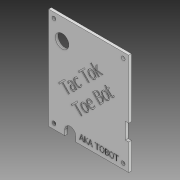
# Autodesk Inventor part: Electronics Lid
Saved by Autodesk Inventor 2020 (Build 240168000, 168)
## iProperties
Created: 2020-09-05
Part Number: Electronics Lid
Material: Generic
Document SubType Name: Modeling
Designer: DDeGo
Density: 1 g/cm^3
Appearance: Default
Author: DDeGo
Autodesk Inventor part; units mm, degrees
ref_plane "YZ Plane" through (0, 0, 0) normal (1, 0, 0) x (0, 1, 0)
ref_plane "XZ Plane" through (0, 0, 0) normal (0, 1, 0) x (-1, 0, 0)
ref_plane "XY Plane" through (0, 0, 0) normal (0, 0, 1) x (1, 0, 0)
sketch "Sketch1" plane through (0, 0, 0) normal (0, 0, 1) x (1, 0, 0)
  line L0 (-37, -47) -> (37, -47)
  line L1 (37, -47) -> (37, 47)
  line L2 (37, 47) -> (-37, 47)
  line L3 (-37, 47) -> (-37, -47)
  line L4 (-37, -47) -> (37, 47) construction
  line L5 (37, -47) -> (-37, 47) construction
  line L6 (-32, -42) -> (32, -42) construction
  line L7 (32, -42) -> (32, 42) construction
  line L8 (32, 42) -> (-32, 42) construction
  line L9 (-32, 42) -> (-32, -42) construction
  line L10 (-32, -42) -> (32, 42) construction
  line L11 (32, -42) -> (-32, 42) construction
  circle A0 centre (-32, 42) radius 1.75
  circle A1 centre (32, 42) radius 1.75
  circle A2 centre (32, -42) radius 1.75
  circle A3 centre (-32, -42) radius 1.75
  point P0 (0, 0)
  dimension "d0" = 74
  dimension "d1" = 94
  dimension "d2" = 84
  dimension "d3" = 64
  dimension "d4" = 3.5
  constraints: 24 end point, 4 centre point, 4 coincident, 4 midpoint, 4 parallel, 3 equal radius, 2 horizontal, 2 perpendicular
  measures "d0" distance of L1.end L2.end
  measures "d1" distance of L0.end L1.end
  measures "d2" distance of L6.end L7.end
  measures "d3" distance of L7.end L8.end
  measures "d4" diameter of A0
extrude "Extrusion1" add sketch "Sketch1" along normal blind 2.5
sketch "Sketch2" plane through (0, 0, 2.5) normal (0, 0, 1) x (1, 0, 0)
  line L0 (37, -47) -> (37, 47) projected
  line L1 (37, -22.5) -> (34, -22.5)
  line L2 (34, -22.5) -> (34, -7.5)
  line L3 (34, -7.5) -> (37, -7.5)
  line L4 (37, -7.5) -> (37, -22.5)
  circle A0 centre (32, -42) radius 1.75 projected
  circle A1 centre (-24.5, 27.5) radius 6.25
  line L5 (37, 47) -> (-37, 47) projected
  line L6 (-37, 47) -> (-37, -47) projected
  arc A2 (-12, -42) -> (-22, -42) centre (-17, -42) ccw
  line L7 (-22, -42) -> (-22, -47)
  line L8 (-37, -47) -> (37, -47) projected
  line L9 (-22, -47) -> (-12, -47)
  line L10 (-12, -47) -> (-12, -42)
  circle A3 centre (-32, -42) radius 1.75 projected
  point P0 (0, 0)
  point P1 (34, -15)
  dimension "d7" = 27
  dimension "d8" = 15
  dimension "d9" = 3
  dimension "d10" = 19.5
  dimension "d11" = 12.5
  dimension "d12" = 12.5
  dimension "d13" = 5
  dimension "d14" = 5
  dimension "d15" = 15
  constraints: 14 end point, 2 centre point, 2 horizontal, 2 parallel, 2 point on circle, 2 point on line, 2 tangent, 2 vertical, 1 midpoint, 1 perpendicular
  measures "d7" vertical distance of A0.centre point (34, -15)
  measures "d8" distance of L1.end L2.end
  measures "d9" distance of L1.start L1.end
  measures "d10" distance from line of L5 A1.centre
  measures "d11" distance from line of L6 A1.centre
  measures "d12" diameter of A1
  measures "d13" radius of A2
  measures "d14" distance from line of L8 A2.centre
  measures "d15" distance of A3.centre A2.centre
extrude "Extrusion2" cut sketch "Sketch2" against normal through all contours L1 L2 L3 L0 | L8 L7 A2 L10 | A0 | A1 | A3
sketch "Sketch3" plane through (0, 0, 2.5) normal (0, 0, 1) x (1, 0, 0)
  line L0 (-28.3077, -7.093) -> (10.2074, 31.4221) construction
  line L1 (10.2074, 31.4221) -> (33.5157, 8.1138) construction
  line L2 (33.5157, 8.1138) -> (-4.9994, -30.4013) construction
  line L3 (-4.9994, -30.4013) -> (-28.3077, -7.093) construction
  line L4 (-12, -47) -> (37, -47) projected
  line L5 (-8.6021, -38.2619) -> (27.6581, -38.2619) construction
  line L6 (27.6581, -38.2619) -> (27.6581, -43.4725) construction
  line L7 (27.6581, -43.4725) -> (-8.6021, -43.4725) construction
  line L8 (-8.6021, -43.4725) -> (-8.6021, -38.2619) construction
  line L9 (-18.5549, -12.1126) -> (-24.7894, -5.8782)
  line L10 (-24.7894, -5.8782) -> (-27.1617, -8.2505)
  line L11 (-27.1617, -8.2505) -> (-27.9983, -7.4139)
  line L12 (-27.9983, -7.4139) -> (-22.3139, -1.7295)
  line L13 (-22.3139, -1.7295) -> (-21.4773, -2.5661)
  line L14 (-21.4773, -2.5661) -> (-23.8496, -4.9384)
  line L15 (-23.8496, -4.9384) -> (-17.6151, -11.1729)
  line L16 (-17.6151, -11.1729) -> (-18.5549, -12.1126)
  spline S0 degree 2 poles (-12.2001, -4.6347) (-12.2288, -4.8238) (-12.309, -5.4771) (-12.3949, -5.7349) knots 0 0 0 1 2 2 2
  spline S1 degree 2 poles (-12.3949, -5.7349) (-12.5038, -6.0959) (-12.8132, -6.6689) (-13.2144, -7.0701) knots 0 0 0 1 2 2 2
  spline S2 degree 2 poles (-13.2144, -7.0701) (-13.541, -7.3967) (-14.3776, -7.7405) (-14.8245, -7.7405) knots 0 0 0 1 2 2 2
  spline S3 degree 2 poles (-14.8245, -7.7405) (-15.2543, -7.7348) (-16.1539, -7.3508) (-16.5092, -6.9956) knots 0 0 0 1 2 2 2
  spline S4 degree 2 poles (-16.5092, -6.9956) (-17.0593, -6.4455) (-17.3745, -5.202) (-17.0937, -4.4743) knots 0 0 0 1 2 2 2
  spline S5 degree 2 poles (-17.0937, -4.4743) (-16.853, -3.821) (-15.7929, -2.4515) (-15.1282, -1.7066) knots 0 0 0 1 2 2 2
  line L17 (-15.1282, -1.7066) -> (-15.3001, -1.5347)
  spline S6 degree 2 poles (-15.3001, -1.5347) (-15.6096, -1.2253) (-16.1826, -1.0304) (-16.4634, -1.0935) knots 0 0 0 1 2 2 2
  spline S7 degree 2 poles (-16.4634, -1.0935) (-16.7442, -1.1565) (-17.3057, -1.5805) (-17.5693, -1.8441) knots 0 0 0 1 2 2 2
  spline S8 degree 2 poles (-17.5693, -1.8441) (-17.8787, -2.1535) (-18.532, -3.1735) (-18.7726, -3.7695) knots 0 0 0 1 2 2 2
  line L18 (-18.7726, -3.7695) -> (-18.8242, -3.821)
  line L19 (-18.8242, -3.821) -> (-19.7353, -2.9099)
  spline S9 degree 2 poles (-19.7353, -2.9099) (-19.5577, -2.5948) (-18.807, -1.5003) (-18.3543, -1.0476) knots 0 0 0 1 2 2 2
  spline S10 degree 2 poles (-18.3543, -1.0476) (-17.8042, -0.4975) (-16.8817, 0.0812) (-16.3602, 0.1557) knots 0 0 0 1 2 2 2
  spline S11 degree 2 poles (-16.3602, 0.1557) (-15.8502, 0.2302) (-14.8704, -0.1766) (-14.3719, -0.6752) knots 0 0 0 1 2 2 2
  line L20 (-14.3719, -0.6752) -> (-10.7446, -4.3024)
  line L21 (-10.7446, -4.3024) -> (-11.6385, -5.1963)
  line L22 (-11.6385, -5.1963) -> (-12.2001, -4.6347)
  line L23 (-12.945, -3.8898) -> (-14.4177, -2.4171)
  spline S12 degree 2 poles (-14.4177, -2.4171) (-14.7099, -2.7667) (-15.5809, -3.8325) (-15.7929, -4.2279) knots 0 0 0 1 2 2 2
  spline S13 degree 2 poles (-15.7929, -4.2279) (-16.0393, -4.692) (-16.0508, -5.6089) (-15.6497, -6.01) knots 0 0 0 1 2 2 2
  spline S14 degree 2 poles (-15.6497, -6.01) (-15.1913, -6.4684) (-14.2114, -6.4168) (-13.7186, -5.924) knots 0 0 0 1 2 2 2
  spline S15 degree 2 poles (-13.7186, -5.924) (-13.3003, -5.5057) (-12.9737, -4.4571) (-12.945, -3.8898) knots 0 0 0 1 2 2 2
  spline S16 degree 2 poles (-7.2607, -1.0591) (-7.8108, -1.6092) (-9.06, -2.1822) (-9.7304, -2.165) knots 0 0 0 1 2 2 2
  spline S17 degree 2 poles (-9.7304, -2.165) (-10.3951, -2.1535) (-11.799, -1.4717) (-12.4981, -0.7726) knots 0 0 0 1 2 2 2
  spline S18 degree 2 poles (-12.4981, -0.7726) (-13.1972, -0.0735) (-13.8447, 1.319) (-13.8733, 1.9779) knots 0 0 0 1 2 2 2
  spline S19 degree 2 poles (-13.8733, 1.9779) (-13.9077, 2.6426) (-13.3461, 3.9491) (-12.8075, 4.4878) knots 0 0 0 1 2 2 2
  spline S20 degree 2 poles (-12.8075, 4.4878) (-12.372, 4.9233) (-11.3119, 5.4905) (-10.8363, 5.6453) knots 0 0 0 1 2 2 2
  line L24 (-10.8363, 5.6453) -> (-9.8335, 4.6425)
  line L25 (-9.8335, 4.6425) -> (-9.8851, 4.5909)
  spline S21 degree 2 poles (-9.8851, 4.5909) (-10.0627, 4.5737) (-10.567, 4.482) (-10.8879, 4.3789) knots 0 0 0 1 2 2 2
  spline S22 degree 2 poles (-10.8879, 4.3789) (-11.1687, 4.2815) (-11.8162, 3.9205) (-12.0454, 3.6913) knots 0 0 0 1 2 2 2
  spline S23 degree 2 poles (-12.0454, 3.6913) (-12.7387, 2.9979) (-12.5325, 1.1069) (-11.5755, 0.15) knots 0 0 0 1 2 2 2
  spline S24 degree 2 poles (-11.5755, 0.15) (-10.6415, -0.784) (-8.7792, -1.019) (-8.0572, -0.297) knots 0 0 0 1 2 2 2
  spline S25 degree 2 poles (-8.0572, -0.297) (-7.6217, 0.1385) (-7.1919, 1.2903) (-7.169, 1.8748) knots 0 0 0 1 2 2 2
  line L26 (-7.169, 1.8748) -> (-7.1174, 1.9264)
  line L27 (-7.1174, 1.9264) -> (-6.1146, 0.9236)
  spline S26 degree 2 poles (-6.1146, 0.9236) (-6.1834, 0.7287) (-6.4069, 0.15) (-6.5272, -0.0506) knots 0 0 0 1 2 2 2
  spline S27 degree 2 poles (-6.5272, -0.0506) (-6.6877, -0.3485) (-6.9799, -0.7783) (-7.2607, -1.0591) knots 0 0 0 1 2 2 2
  line L28 (-0.2469, 6.1954) -> (-6.4814, 12.4298)
  line L29 (-6.4814, 12.4298) -> (-8.8537, 10.0575)
  line L30 (-8.8537, 10.0575) -> (-9.6903, 10.8941)
  line L31 (-9.6903, 10.8941) -> (-4.0059, 16.5785)
  line L32 (-4.0059, 16.5785) -> (-3.1693, 15.7419)
  line L33 (-3.1693, 15.7419) -> (-5.5416, 13.3696)
  line L34 (-5.5416, 13.3696) -> (0.6928, 7.1351)
  line L35 (0.6928, 7.1351) -> (-0.2469, 6.1954)
  spline S28 degree 2 poles (5.4203, 17.1687) (6.7611, 15.8278) (6.933, 13.0773) (5.8558, 12) knots 0 0 0 1 2 2 2
  spline S29 degree 2 poles (5.8558, 12) (4.7498, 10.8941) (1.9764, 11.1348) (0.6814, 12.4298) knots 0 0 0 1 2 2 2
  spline S30 degree 2 poles (0.6814, 12.4298) (-0.648, 13.7592) (-0.8142, 16.5384) (0.2516, 17.6042) knots 0 0 0 1 2 2 2
  spline S31 degree 2 poles (0.2516, 17.6042) (1.3289, 18.6815) (4.0851, 18.5038) (5.4203, 17.1687) knots 0 0 0 1 2 2 2
  spline S32 degree 2 poles (4.4977, 16.2461) (3.4663, 17.2776) (1.7128, 17.5297) (1.0195, 16.8363) knots 0 0 0 1 2 2 2
  spline S33 degree 2 poles (1.0195, 16.8363) (0.3261, 16.143) (0.5725, 14.3838) (1.6039, 13.3524) knots 0 0 0 1 2 2 2
  spline S34 degree 2 poles (1.6039, 13.3524) (2.6067, 12.3496) (4.3946, 12.0745) (5.0879, 12.7679) knots 0 0 0 1 2 2 2
  spline S35 degree 2 poles (5.0879, 12.7679) (5.7755, 13.4555) (5.5177, 15.2262) (4.4977, 16.2461) knots 0 0 0 1 2 2 2
  line L36 (13.3852, 19.8275) -> (12.2105, 18.6528)
  line L37 (12.2105, 18.6528) -> (7.678, 19.243)
  line L38 (7.678, 19.243) -> (7.6665, 18.5439)
  line L39 (7.6665, 18.5439) -> (9.8841, 16.3264)
  line L40 (9.8841, 16.3264) -> (8.9902, 15.4324)
  line L41 (8.9902, 15.4324) -> (1.6039, 22.8187)
  line L42 (1.6039, 22.8187) -> (2.4979, 23.7126)
  line L43 (2.4979, 23.7126) -> (6.8184, 19.392)
  line L44 (6.8184, 19.392) -> (6.6752, 23.7298)
  line L45 (6.6752, 23.7298) -> (7.7868, 24.8414)
  line L46 (7.7868, 24.8414) -> (7.8269, 20.4464)
  line L47 (7.8269, 20.4464) -> (13.3852, 19.8275)
  line L48 (-6.9126, -23.755) -> (-13.147, -17.5205)
  line L49 (-13.147, -17.5205) -> (-15.5193, -19.8928)
  line L50 (-15.5193, -19.8928) -> (-16.3559, -19.0562)
  line L51 (-16.3559, -19.0562) -> (-10.6716, -13.3718)
  line L52 (-10.6716, -13.3718) -> (-9.835, -14.2084)
  line L53 (-9.835, -14.2084) -> (-12.2073, -16.5808)
  line L54 (-12.2073, -16.5808) -> (-5.9728, -22.8152)
  line L55 (-5.9728, -22.8152) -> (-6.9126, -23.755)
  spline S36 degree 2 poles (-1.2454, -12.7816) (0.0955, -14.1225) (0.2674, -16.873) (-0.8099, -17.9503) knots 0 0 0 1 2 2 2
  spline S37 degree 2 poles (-0.8099, -17.9503) (-1.9158, -19.0562) (-4.6893, -18.8155) (-5.9843, -17.5205) knots 0 0 0 1 2 2 2
  spline S38 degree 2 poles (-5.9843, -17.5205) (-7.3137, -16.1911) (-7.4799, -13.412) (-6.414, -12.3461) knots 0 0 0 1 2 2 2
  spline S39 degree 2 poles (-6.414, -12.3461) (-5.3368, -11.2689) (-2.5805, -11.4465) (-1.2454, -12.7816) knots 0 0 0 1 2 2 2
  spline S40 degree 2 poles (-2.168, -13.7042) (-3.1994, -12.6728) (-4.9528, -12.4206) (-5.6462, -13.114) knots 0 0 0 1 2 2 2
  spline S41 degree 2 poles (-5.6462, -13.114) (-6.3396, -13.8073) (-6.0932, -15.5665) (-5.0617, -16.5979) knots 0 0 0 1 2 2 2
  spline S42 degree 2 poles (-5.0617, -16.5979) (-4.0589, -17.6007) (-2.2711, -17.8758) (-1.5778, -17.1824) knots 0 0 0 1 2 2 2
  spline S43 degree 2 poles (-1.5778, -17.1824) (-0.8901, -16.4948) (-1.148, -14.7242) (-2.168, -13.7042) knots 0 0 0 1 2 2 2
  spline S44 degree 2 poles (4.7484, -12.3347) (3.4763, -13.6068) (0.6513, -13.5781) (-0.6667, -12.2602) knots 0 0 0 1 2 2 2
  spline S45 degree 2 poles (-0.6667, -12.2602) (-1.9617, -10.9652) (-2.1393, -8.0714) (-1.0448, -6.9769) knots 0 0 0 1 2 2 2
  spline S46 degree 2 poles (-1.0448, -6.9769) (-0.5521, -6.4841) (0.4966, -6.0085) (1.0811, -6.0315) knots 0 0 0 1 2 2 2
  spline S47 degree 2 poles (1.0811, -6.0315) (1.6713, -6.0486) (2.8517, -6.6217) (3.4877, -7.2577) knots 0 0 0 1 2 2 2
  line L56 (3.4877, -7.2577) -> (3.9748, -7.7448)
  line L57 (3.9748, -7.7448) -> (0.3017, -11.4178)
  spline S48 degree 2 poles (0.3017, -11.4178) (1.2243, -12.3404) (3.1325, -12.392) (3.9576, -11.5668) knots 0 0 0 1 2 2 2
  spline S49 degree 2 poles (3.9576, -11.5668) (4.2499, -11.2746) (4.6854, -10.5755) (4.8114, -10.2431) knots 0 0 0 1 2 2 2
  spline S50 degree 2 poles (4.8114, -10.2431) (4.9375, -9.8879) (5.0693, -9.355) (5.0865, -9.1544) knots 0 0 0 1 2 2 2
  line L58 (5.0865, -9.1544) -> (5.138, -9.1028)
  line L59 (5.138, -9.1028) -> (6.1122, -10.077)
  spline S51 degree 2 poles (6.1122, -10.077) (6.0205, -10.2947) (5.734, -10.948) (5.6022, -11.1829) knots 0 0 0 1 2 2 2
  spline S52 degree 2 poles (5.6022, -11.1829) (5.4188, -11.5153) (5.0693, -12.0138) (4.7484, -12.3347) knots 0 0 0 1 2 2 2
  spline S53 degree 2 poles (2.4219, -7.9339) (2.0495, -7.5843) (1.3733, -7.2061) (1.0524, -7.1718) knots 0 0 0 1 2 2 2
  spline S54 degree 2 poles (1.0524, -7.1718) (0.6971, -7.1259) (-0.002, -7.401) (-0.363, -7.762) knots 0 0 0 1 2 2 2
  spline S55 degree 2 poles (-0.363, -7.762) (-0.7182, -8.1172) (-1.0047, -8.8278) (-1.0047, -9.2404) knots 0 0 0 1 2 2 2
  spline S56 degree 2 poles (-1.0047, -9.2404) (-0.9933, -9.6529) (-0.6896, -10.3692) (-0.3801, -10.7359) knots 0 0 0 1 2 2 2
  line L60 (-0.3801, -10.7359) -> (2.4219, -7.9339)
  spline S57 degree 2 poles (13.1718, 0.6729) (13.699, 0.1457) (14.1058, -1.0634) (14.037, -1.6593) knots 0 0 0 1 2 2 2
  spline S58 degree 2 poles (14.037, -1.6593) (13.9454, -2.3699) (13.2978, -3.5445) (12.5758, -4.2665) knots 0 0 0 1 2 2 2
  line L61 (12.5758, -4.2665) -> (10.5473, -6.295)
  line L62 (10.5473, -6.295) -> (3.4763, 0.776)
  line L63 (3.4763, 0.776) -> (5.3501, 2.6498)
  spline S59 degree 2 poles (5.3501, 2.6498) (6.1064, 3.4062) (6.9602, 4.0652) (7.4932, 4.2199) knots 0 0 0 1 2 2 2
  spline S60 degree 2 poles (7.4932, 4.2199) (8.0776, 4.4032) (9.0861, 4.0938) (9.5331, 3.6469) knots 0 0 0 1 2 2 2
  spline S61 degree 2 poles (9.5331, 3.6469) (10.0316, 3.1483) (10.2952, 1.8304) (10.0546, 1.1428) knots 0 0 0 1 2 2 2
  line L64 (10.0546, 1.1428) -> (10.0889, 1.1084)
  spline S62 degree 2 poles (10.0889, 1.1084) (10.8912, 1.5668) (12.4956, 1.349) (13.1718, 0.6729) knots 0 0 0 1 2 2 2
  spline S63 degree 2 poles (12.232, -0.3471) (11.8309, 0.054) (11.086, 0.3405) (10.5588, 0.1801) knots 0 0 0 1 2 2 2
  spline S64 degree 2 poles (10.5588, 0.1801) (10.2207, 0.0712) (9.6248, -0.3872) (9.1377, -0.8743) knots 0 0 0 1 2 2 2
  line L65 (9.1377, -0.8743) -> (8.0719, -1.9401)
  line L66 (8.0719, -1.9401) -> (10.6849, -4.5531)
  line L67 (10.6849, -4.5531) -> (11.447, -3.7909)
  spline S65 degree 2 poles (11.447, -3.7909) (12.0659, -3.1721) (12.6618, -2.3469) (12.7535, -1.8885) knots 0 0 0 1 2 2 2
  spline S66 degree 2 poles (12.7535, -1.8885) (12.828, -1.4358) (12.6045, -0.7196) (12.232, -0.3471) knots 0 0 0 1 2 2 2
  spline S67 degree 2 poles (8.685, 2.5352) (8.4329, 2.7873) (7.8828, 2.9936) (7.5848, 2.9134) knots 0 0 0 1 2 2 2
  spline S68 degree 2 poles (7.5848, 2.9134) (7.2296, 2.8102) (6.6164, 2.3117) (6.1179, 1.8132) knots 0 0 0 1 2 2 2
  line L68 (6.1179, 1.8132) -> (5.2183, 0.9136)
  line L69 (5.2183, 0.9136) -> (7.2869, -1.1551)
  line L70 (7.2869, -1.1551) -> (8.3527, -0.0892)
  spline S69 degree 2 poles (8.3527, -0.0892) (8.7939, 0.352) (9.1205, 0.862) (9.2008, 1.2287) knots 0 0 0 1 2 2 2
  spline S70 degree 2 poles (9.2008, 1.2287) (9.281, 1.584) (9.0174, 2.2028) (8.685, 2.5352) knots 0 0 0 1 2 2 2
  spline S71 degree 2 poles (17.9164, 6.3802) (19.2573, 5.0393) (19.4292, 2.2888) (18.3519, 1.2115) knots 0 0 0 1 2 2 2
  spline S72 degree 2 poles (18.3519, 1.2115) (17.246, 0.1056) (14.4725, 0.3463) (13.1775, 1.6413) knots 0 0 0 1 2 2 2
  spline S73 degree 2 poles (13.1775, 1.6413) (11.8481, 2.9707) (11.6819, 5.7498) (12.7477, 6.8157) knots 0 0 0 1 2 2 2
  spline S74 degree 2 poles (12.7477, 6.8157) (13.825, 7.8929) (16.5812, 7.7153) (17.9164, 6.3802) knots 0 0 0 1 2 2 2
  spline S75 degree 2 poles (16.9938, 5.4576) (15.9624, 6.489) (14.2089, 6.7412) (13.5156, 6.0478) knots 0 0 0 1 2 2 2
  spline S76 degree 2 poles (13.5156, 6.0478) (12.8222, 5.3545) (13.0686, 3.5953) (14.1001, 2.5638) knots 0 0 0 1 2 2 2
  spline S77 degree 2 poles (14.1001, 2.5638) (15.1029, 1.5611) (16.8907, 1.286) (17.584, 1.9794) knots 0 0 0 1 2 2 2
  spline S78 degree 2 poles (17.584, 1.9794) (18.2717, 2.667) (18.0138, 4.4376) (16.9938, 5.4576) knots 0 0 0 1 2 2 2
  spline S79 degree 2 poles (23.1939, 6.1452) (22.4662, 5.4175) (20.8159, 5.429) (19.9162, 6.3286) knots 0 0 0 1 2 2 2
  line L71 (19.9162, 6.3286) -> (16.9766, 9.2682)
  line L72 (16.9766, 9.2682) -> (16.375, 8.6665)
  line L73 (16.375, 8.6665) -> (15.6358, 9.4057)
  line L74 (15.6358, 9.4057) -> (16.2374, 10.0074)
  line L75 (16.2374, 10.0074) -> (14.7132, 11.5316)
  line L76 (14.7132, 11.5316) -> (15.6071, 12.4255)
  line L77 (15.6071, 12.4255) -> (17.1313, 10.9013)
  line L78 (17.1313, 10.9013) -> (18.7759, 12.5459)
  line L79 (18.7759, 12.5459) -> (19.5151, 11.8067)
  line L80 (19.5151, 11.8067) -> (17.8705, 10.1621)
  line L81 (17.8705, 10.1621) -> (20.3976, 7.6351)
  spline S80 degree 2 poles (20.3976, 7.6351) (20.7987, 7.234) (21.2686, 6.8214) (21.5551, 6.7297) knots 0 0 0 1 2 2 2
  spline S81 degree 2 poles (21.5551, 6.7297) (21.8015, 6.6438) (22.3286, 6.8386) (22.6381, 7.148) knots 0 0 0 1 2 2 2
  spline S82 degree 2 poles (22.6381, 7.148) (22.8558, 7.3658) (23.1309, 7.9044) (23.1824, 8.0362) knots 0 0 0 1 2 2 2
  line L82 (23.1824, 8.0362) -> (23.234, 8.0878)
  line L83 (23.234, 8.0878) -> (24.0362, 7.2855)
  spline S83 degree 2 poles (24.0362, 7.2855) (23.8529, 6.9646) (23.4174, 6.3687) (23.1939, 6.1452) knots 0 0 0 1 2 2 2
  line L84 (-8.6345, -43.3672) -> (-6.9489, -38.3672)
  line L85 (-6.9489, -38.3672) -> (-6.1304, -38.3672)
  line L86 (-6.1304, -38.3672) -> (-4.4448, -43.3672)
  line L87 (-4.4448, -43.3672) -> (-5.1458, -43.3672)
  line L88 (-5.1458, -43.3672) -> (-5.5996, -41.9693)
  line L89 (-5.5996, -41.9693) -> (-7.5081, -41.9693)
  line L90 (-7.5081, -41.9693) -> (-7.9619, -43.3672)
  line L91 (-7.9619, -43.3672) -> (-8.6345, -43.3672)
  line L92 (-5.782, -41.402) -> (-6.5559, -39.0479)
  line L93 (-6.5559, -39.0479) -> (-7.3257, -41.402)
  line L94 (-7.3257, -41.402) -> (-5.782, -41.402)
  line L95 (-0.3241, -43.3672) -> (-1.1871, -43.3672)
  line L96 (-1.1871, -43.3672) -> (-3.0145, -41.0414)
  line L97 (-3.0145, -41.0414) -> (-3.3063, -41.3696)
  line L98 (-3.3063, -41.3696) -> (-3.3063, -43.3672)
  line L99 (-3.3063, -43.3672) -> (-3.9708, -43.3672)
  line L100 (-3.9708, -43.3672) -> (-3.9708, -38.3672)
  line L101 (-3.9708, -38.3672) -> (-3.3063, -38.3672)
  line L102 (-3.3063, -38.3672) -> (-3.3063, -40.6646)
  line L103 (-3.3063, -40.6646) -> (-1.256, -38.3672)
  line L104 (-1.256, -38.3672) -> (-0.4457, -38.3672)
  line L105 (-0.4457, -38.3672) -> (-2.5162, -40.5998)
  line L106 (-2.5162, -40.5998) -> (-0.3241, -43.3672)
  line L107 (-0.4659, -43.3672) -> (1.2197, -38.3672)
  line L108 (1.2197, -38.3672) -> (2.0381, -38.3672)
  line L109 (2.0381, -38.3672) -> (3.7237, -43.3672)
  line L110 (3.7237, -43.3672) -> (3.0227, -43.3672)
  line L111 (3.0227, -43.3672) -> (2.5689, -41.9693)
  line L112 (2.5689, -41.9693) -> (0.6605, -41.9693)
  line L113 (0.6605, -41.9693) -> (0.2067, -43.3672)
  line L114 (0.2067, -43.3672) -> (-0.4659, -43.3672)
  line L115 (2.3866, -41.402) -> (1.6127, -39.0479)
  line L116 (1.6127, -39.0479) -> (0.8428, -41.402)
  line L117 (0.8428, -41.402) -> (2.3866, -41.402)
  line L118 (7.5122, -43.3672) -> (7.5122, -38.9588)
  line L119 (7.5122, -38.9588) -> (5.8347, -38.9588)
  line L120 (5.8347, -38.9588) -> (5.8347, -38.3672)
  line L121 (5.8347, -38.3672) -> (9.8542, -38.3672)
  line L122 (9.8542, -38.3672) -> (9.8542, -38.9588)
  line L123 (9.8542, -38.9588) -> (8.1767, -38.9588)
  line L124 (8.1767, -38.9588) -> (8.1767, -43.3672)
  line L125 (8.1767, -43.3672) -> (7.5122, -43.3672)
  spline S84 degree 2 poles (13.8979, -38.9385) (14.1816, -39.2708) (14.4976, -40.2432) (14.4976, -40.8672) knots 0 0 0 1 2 2 2
  spline S85 degree 2 poles (14.4976, -40.8672) (14.4976, -41.475) (14.1897, -42.4596) (13.8979, -42.7918) knots 0 0 0 1 2 2 2
  spline S86 degree 2 poles (13.8979, -42.7918) (13.59, -43.1403) (12.7756, -43.4725) (12.2853, -43.4725) knots 0 0 0 1 2 2 2
  spline S87 degree 2 poles (12.2853, -43.4725) (11.7788, -43.4725) (10.9684, -43.1281) (10.6727, -42.7918) knots 0 0 0 1 2 2 2
  spline S88 degree 2 poles (10.6727, -42.7918) (10.385, -42.4596) (10.077, -41.4831) (10.077, -40.8672) knots 0 0 0 1 2 2 2
  spline S89 degree 2 poles (10.077, -40.8672) (10.077, -40.2392) (10.389, -39.2829) (10.6767, -38.9385) knots 0 0 0 1 2 2 2
  spline S90 degree 2 poles (10.6767, -38.9385) (10.9684, -38.6063) (11.7829, -38.2619) (12.2853, -38.2619) knots 0 0 0 1 2 2 2
  spline S91 degree 2 poles (12.2853, -38.2619) (12.7958, -38.2619) (13.6143, -38.6184) (13.8979, -38.9385) knots 0 0 0 1 2 2 2
  spline S92 degree 2 poles (13.8048, -40.8672) (13.8048, -40.3729) (13.59, -39.6071) (13.3955, -39.3559) knots 0 0 0 1 2 2 2
  spline S93 degree 2 poles (13.3955, -39.3559) (13.197, -39.0965) (12.6378, -38.8372) (12.2894, -38.8372) knots 0 0 0 1 2 2 2
  spline S94 degree 2 poles (12.2894, -38.8372) (11.9287, -38.8372) (11.3858, -39.0884) (11.1791, -39.3559) knots 0 0 0 1 2 2 2
  spline S95 degree 2 poles (11.1791, -39.3559) (10.9806, -39.6111) (10.7699, -40.381) (10.7699, -40.8672) knots 0 0 0 1 2 2 2
  spline S96 degree 2 poles (10.7699, -40.8672) (10.7699, -41.8518) (11.5965, -42.8972) (12.2894, -42.8972) knots 0 0 0 1 2 2 2
  spline S97 degree 2 poles (12.2894, -42.8972) (12.9822, -42.8972) (13.8048, -41.8518) (13.8048, -40.8672) knots 0 0 0 1 2 2 2
  spline S98 degree 2 poles (18.6184, -41.8315) (18.6184, -42.2043) (18.3347, -42.7756) (18.0997, -42.962) knots 0 0 0 1 2 2 2
  spline S99 degree 2 poles (18.0997, -42.962) (17.8161, -43.1808) (17.1718, -43.3672) (16.6613, -43.3672) knots 0 0 0 1 2 2 2
  line L126 (16.6613, -43.3672) -> (15.227, -43.3672)
  line L127 (15.227, -43.3672) -> (15.227, -38.3672)
  line L128 (15.227, -38.3672) -> (16.5519, -38.3672)
  spline S100 degree 2 poles (16.5519, -38.3672) (17.0868, -38.3672) (17.6216, -38.4361) (17.8647, -38.5698) knots 0 0 0 1 2 2 2
  spline S101 degree 2 poles (17.8647, -38.5698) (18.1362, -38.7116) (18.3834, -39.1776) (18.3834, -39.4936) knots 0 0 0 1 2 2 2
  spline S102 degree 2 poles (18.3834, -39.4936) (18.3834, -39.8461) (18.0106, -40.4053) (17.6824, -40.5633) knots 0 0 0 1 2 2 2
  line L129 (17.6824, -40.5633) -> (17.6824, -40.5876)
  spline S103 degree 2 poles (17.6824, -40.5876) (18.1281, -40.7092) (18.6184, -41.3534) (18.6184, -41.8315) knots 0 0 0 1 2 2 2
  spline S104 degree 2 poles (17.9255, -41.8599) (17.9255, -41.5763) (17.7634, -41.2116) (17.5203, -41.0819) knots 0 0 0 1 2 2 2
  spline S105 degree 2 poles (17.5203, -41.0819) (17.3623, -41.0009) (16.9895, -40.9523) (16.6451, -40.9523) knots 0 0 0 1 2 2 2
  line L130 (16.6451, -40.9523) -> (15.8915, -40.9523)
  line L131 (15.8915, -40.9523) -> (15.8915, -42.7999)
  line L132 (15.8915, -42.7999) -> (16.4304, -42.7999)
  spline S106 degree 2 poles (16.4304, -42.7999) (16.868, -42.7999) (17.3704, -42.7189) (17.5649, -42.5892) knots 0 0 0 1 2 2 2
  spline S107 degree 2 poles (17.5649, -42.5892) (17.7513, -42.4555) (17.9255, -42.1233) (17.9255, -41.8599) knots 0 0 0 1 2 2 2
  spline S108 degree 2 poles (17.6905, -39.5868) (17.6905, -39.4085) (17.5689, -39.1411) (17.4352, -39.0641) knots 0 0 0 1 2 2 2
  spline S109 degree 2 poles (17.4352, -39.0641) (17.2731, -38.975) (16.8801, -38.9345) (16.5276, -38.9345) knots 0 0 0 1 2 2 2
  line L133 (16.5276, -38.9345) -> (15.8915, -38.9345)
  line L134 (15.8915, -38.9345) -> (15.8915, -40.3972)
  line L135 (15.8915, -40.3972) -> (16.6451, -40.3972)
  spline S110 degree 2 poles (16.6451, -40.3972) (16.9571, -40.3972) (17.2529, -40.3324) (17.4109, -40.2311) knots 0 0 0 1 2 2 2
  spline S111 degree 2 poles (17.4109, -40.2311) (17.5649, -40.1338) (17.6905, -39.8218) (17.6905, -39.5868) knots 0 0 0 1 2 2 2
  spline S112 degree 2 poles (22.8161, -38.9385) (23.0997, -39.2708) (23.4158, -40.2432) (23.4158, -40.8672) knots 0 0 0 1 2 2 2
  spline S113 degree 2 poles (23.4158, -40.8672) (23.4158, -41.475) (23.1078, -42.4596) (22.8161, -42.7918) knots 0 0 0 1 2 2 2
  spline S114 degree 2 poles (22.8161, -42.7918) (22.5082, -43.1403) (21.6937, -43.4725) (21.2035, -43.4725) knots 0 0 0 1 2 2 2
  spline S115 degree 2 poles (21.2035, -43.4725) (20.697, -43.4725) (19.8866, -43.1281) (19.5908, -42.7918) knots 0 0 0 1 2 2 2
  spline S116 degree 2 poles (19.5908, -42.7918) (19.3031, -42.4596) (18.9952, -41.4831) (18.9952, -40.8672) knots 0 0 0 1 2 2 2
  spline S117 degree 2 poles (18.9952, -40.8672) (18.9952, -40.2392) (19.3072, -39.2829) (19.5949, -38.9385) knots 0 0 0 1 2 2 2
  spline S118 degree 2 poles (19.5949, -38.9385) (19.8866, -38.6063) (20.701, -38.2619) (21.2035, -38.2619) knots 0 0 0 1 2 2 2
  spline S119 degree 2 poles (21.2035, -38.2619) (21.714, -38.2619) (22.5325, -38.6184) (22.8161, -38.9385) knots 0 0 0 1 2 2 2
  spline S120 degree 2 poles (22.7229, -40.8672) (22.7229, -40.3729) (22.5082, -39.6071) (22.3137, -39.3559) knots 0 0 0 1 2 2 2
  spline S121 degree 2 poles (22.3137, -39.3559) (22.1151, -39.0965) (21.556, -38.8372) (21.2075, -38.8372) knots 0 0 0 1 2 2 2
  spline S122 degree 2 poles (21.2075, -38.8372) (20.8469, -38.8372) (20.3039, -39.0884) (20.0973, -39.3559) knots 0 0 0 1 2 2 2
  spline S123 degree 2 poles (20.0973, -39.3559) (19.8988, -39.6111) (19.6881, -40.381) (19.6881, -40.8672) knots 0 0 0 1 2 2 2
  spline S124 degree 2 poles (19.6881, -40.8672) (19.6881, -41.8518) (20.5146, -42.8972) (21.2075, -42.8972) knots 0 0 0 1 2 2 2
  spline S125 degree 2 poles (21.2075, -42.8972) (21.9004, -42.8972) (22.7229, -41.8518) (22.7229, -40.8672) knots 0 0 0 1 2 2 2
  line L136 (25.312, -43.3672) -> (25.312, -38.9588)
  line L137 (25.312, -38.9588) -> (23.6346, -38.9588)
  line L138 (23.6346, -38.9588) -> (23.6346, -38.3672)
  line L139 (23.6346, -38.3672) -> (27.654, -38.3672)
  line L140 (27.654, -38.3672) -> (27.654, -38.9588)
  line L141 (27.654, -38.9588) -> (25.9765, -38.9588)
  line L142 (25.9765, -38.9588) -> (25.9765, -43.3672)
  line L143 (25.9765, -43.3672) -> (25.312, -43.3672)
  point P0 (0, 0)
  dimension "d20" = 45
  constraints: 4 other
  measures "d20" angle of L4 L2
extrude "Extrusion3" cut sketch "Sketch3" against normal blind 0.5
body "Solid1"
